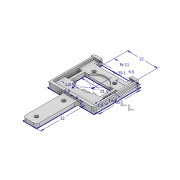
# Autodesk Inventor part: Intan_holder_test_main
Saved by Autodesk Inventor 2020 (Build 240168000, 168)
## iProperties
Created: 2020-07-20
Part Number: Intan_holder_test_main
Material: Generic
Document SubType Name: Modeling
Designer: Daniel
Density: 1 g/cm^3
Appearance: Default
Author: Daniel
Autodesk Inventor part; units mm, degrees
ref_plane "YZ Plane" through (0, 0, 0) normal (1, 0, 0) x (0, 1, 0)
ref_plane "XZ Plane" through (0, 0, 0) normal (0, 1, 0) x (-1, 0, 0)
ref_plane "XY Plane" through (0, 0, 0) normal (0, 0, 1) x (1, 0, 0)
sketch "Sketch1" plane through (0, 0, 0) normal (0, 1, 0) x (-1, 0, 0)
  line L0 (5, 16) -> (-5, 16)
  line L1 (-5, 16) -> (-5, -16)
  line L2 (-5, -16) -> (5, -16)
  line L3 (5, -16) -> (5, 16)
  line L4 (5, 16) -> (-5, -16) construction
  line L5 (-5, 16) -> (5, -16) construction
  line L6 (15.05, -16) -> (-15.05, -16)
  line L7 (-15.05, -16) -> (-15.05, -46.1)
  line L8 (-15.05, -46.1) -> (15.05, -46.1)
  line L9 (15.05, -46.1) -> (15.05, -16)
  line L10 (15.05, -16) -> (-15.05, -46.1) construction
  line L11 (-15.05, -16) -> (15.05, -46.1) construction
  line L12 (-17.05, -48.1) -> (-17.05, -14)
  line L13 (-17.05, -14) -> (17.05, -14)
  line L14 (17.05, -14) -> (17.05, -48.1)
  line L15 (17.05, -48.1) -> (-17.05, -48.1)
  line L16 (-11, -43.6) -> (11, -43.6)
  line L17 (10.55, -34.9) -> (-10.55, -34.9)
  line L18 (10.55, -24.8) -> (-10.55, -24.8)
  line L19 (10.55, -34.9) -> (-10.55, -34.9) construction
  line L20 (-10.55, -34.9) -> (-10.55, -24.8) construction
  line L21 (-10.55, -24.8) -> (10.55, -24.8)
  line L22 (10.55, -24.8) -> (10.55, -34.9) construction
  line L23 (10.55, -34.9) -> (-10.55, -24.8) construction
  line L24 (-10.55, -34.9) -> (10.55, -24.8) construction
  line L25 (10.55, -24.8) -> (10.55, -34.9)
  line L26 (-10.55, -24.8) -> (-10.55, -34.9)
  line L27 (-11, -43.6) -> (-11, -48.1)
  line L28 (11, -43.6) -> (11, -48.1)
  line L29 (15.05, -24.8) -> (12.35, -24.8)
  line L30 (12.35, -24.8) -> (12.35, -34.9)
  line L31 (12.35, -34.9) -> (15.05, -34.9)
  line L32 (15.05, -34.9) -> (15.05, -24.8)
  line L33 (-15.05, -24.8) -> (-12.35, -24.8)
  line L34 (-12.35, -24.8) -> (-12.35, -34.9)
  line L35 (-12.35, -34.9) -> (-15.05, -34.9)
  line L36 (-15.05, -34.9) -> (-15.05, -24.8)
  point P0 (0, 0)
  point P1 (0, -31.05)
  point P2 (0, 0)
  point P3 (0, -31.05)
  point P4 (0, -29.85)
  point P5 (0, -29.85)
  point P6 (0, -31.05)
  point P7 (5, -14)
  point P8 (-5, -14)
  point P9 (5, -16)
  point P10 (-5, -16)
  point P11 (-11, -46.1)
  point P12 (11, -46.1)
  point P13 (-15.05, -34.9)
  dimension "d19" = 10
  dimension "d20" = 32
  dimension "d23" = 30.1
  dimension "d24" = 30.1
  dimension "d26" = 2
  dimension "d29" = 4.5
  dimension "d31" = 8.8
  dimension "d32" = 21.1
  dimension "d33" = 10.1
  dimension "d37" = 22
  dimension "d38" = 11
  dimension "d132" = 1.8
  dimension "d133" = 1.8
  constraints: 74 end point, 12 parallel, 11 perpendicular, 10 midpoint, 7 point on line, 5 collinear, 5 horizontal, 2 vertical alignment, 3 other
  measures "d19" distance of L2.end L1.end
  measures "d20" distance of L1.end L0.end
  measures "d23" distance of L8.end L7.end
  measures "d24" distance of L7.end L6.end
  measures "d26" distance between parallel lines of L7 L12
  measures "d29" distance between parallel lines of L15 L16
  measures "d31" distance between parallel lines of L6 L18
  measures "d32" distance of L18.start L18.end
  measures "d33" distance of L18.end L19.end
  measures "d37" distance between parallel lines of L27 L28
  measures "d38" distance from line of point (0, -31.05) L28
  measures "d132" distance between parallel lines of L22 L30
  measures "d133" distance between parallel lines of L20 L34
extrude "Base" add sketch "Sketch1" along normal blind 2.6 contours L3 L13 L1 L0 | L3 L2 L1 L13 | L6 L9 L29 L30 L31 L8 L28 L16 L27 L7 L35 L34 L33 L2
extrude "Adaptor board recess" add sketch "Sketch1" along normal blind 4.2 contours L13 L14 L15 L28 L8 L9 L6 L3 | L3 L2 L1 L13 | L1 L6 L7 L8 L27 L15 L12 L13
sketch "Sketch3" plane through (0, 2.6, 0) normal (0, 1, 0) x (1, 0, 0)
  circle A0 centre (0, 31.05) radius 8.75
  line L0 (15.05, 16) -> (-15.05, 16) projected
  line L1 (-15.05, 16) -> (15.05, 16) projected
  line L2 (15.05, 34.9) -> (15.05, 46.1) projected
  line L3 (15.05, 46.1) -> (11, 46.1) projected
  line L4 (11, 46.1) -> (11, 43.6) projected
  line L5 (11, 43.6) -> (-11, 43.6) projected
  line L6 (-11, 43.6) -> (-11, 46.1) projected
  line L7 (-11, 46.1) -> (-15.05, 46.1) projected
  line L8 (-15.05, 46.1) -> (-15.05, 34.9) projected
  line L9 (10.55, 34.9) -> (10.55, 24.8) projected
  line L10 (10.55, 24.8) -> (-10.55, 24.8) projected
  line L11 (-10.55, 24.8) -> (-10.55, 34.9) projected
  line L12 (-10.55, 34.9) -> (10.55, 34.9) projected
  line L13 (15.05, 16) -> (15.05, 24.8) projected
  line L14 (15.05, 24.8) -> (12.35, 24.8) projected
  line L15 (12.35, 24.8) -> (12.35, 34.9) projected
  line L16 (12.35, 34.9) -> (15.05, 34.9) projected
  line L17 (-15.05, 34.9) -> (-12.35, 34.9) projected
  line L18 (-12.35, 34.9) -> (-12.35, 24.8) projected
  line L19 (-12.35, 24.8) -> (-15.05, 24.8) projected
  line L20 (-15.05, 24.8) -> (-15.05, 16) projected
  point P0 (0, 0)
  point P1 (0, 16)
  point P2 (-17.25, 14.5)
  point P3 (17.25, 14.5)
  point P4 (-9.5909, 26.1961)
  point P5 (9.5909, 26.1961)
  point P6 (6.1237, 24.8)
  point P7 (-6.1237, 24.8)
  point P8 (7.8575, 34.9)
  point P9 (9.5909, 31.858)
  point P10 (-9.5909, 31.858)
  point P11 (-7.8575, 34.9)
  dimension "d39" = 17.5
  constraints: 1 centre point, 1 coincident, 1 midpoint, 1 vertical alignment
  measures "d39" diameter of A0
extrude "EIB recess" cut sketch "Sketch3" against normal blind 1 contours L12 A0 | A0 L10
sketch "Sketch4" plane through (0, 2.6, 0) normal (0, 1, 0) x (1, 0, 0)
  circle A0 centre (7.5, 38.6) radius 1.3
  circle A1 centre (-7.5, 38.6) radius 1.3
  line L0 (5.9412, 41.3) -> (9.0588, 41.3)
  line L1 (9.0588, 41.3) -> (10.6177, 38.6)
  line L2 (10.6177, 38.6) -> (9.0588, 35.9)
  line L3 (9.0588, 35.9) -> (5.9412, 35.9)
  line L4 (5.9412, 35.9) -> (4.3823, 38.6)
  line L5 (4.3823, 38.6) -> (5.9412, 41.3)
  line L6 (-10.6177, 38.6) -> (-9.0588, 41.3)
  line L7 (-9.0588, 41.3) -> (-5.9412, 41.3)
  line L8 (-5.9412, 41.3) -> (-4.3823, 38.6)
  line L9 (-4.3823, 38.6) -> (-5.9412, 35.9)
  line L10 (-5.9412, 35.9) -> (-9.0588, 35.9)
  line L11 (-9.0588, 35.9) -> (-10.6177, 38.6)
  line L12 (11, 43.6) -> (-11, 43.6) construction
  point P0 (0, 0)
  dimension "d42" = 2.6
  dimension "d43" = 2.6
  dimension "d45" = 15
  dimension "d46" = 7.5
  dimension "d57" = 5.4
  dimension "d58" = 5.4
  dimension "d127" = 2.3
  constraints: 24 end point, 2 centre point, 2 coincident, 2 horizontal, 1 horizontal alignment, 26 other
  measures "d42" diameter of A0
  measures "d43" diameter of A1
  measures "d45" distance of A1.centre A0.centre
  measures "d46" horizontal distance of point (0, 0) A1.centre
  measures "d57" distance between parallel lines of L3 L0
  measures "d58" distance between parallel lines of L10 L7
  measures "d127" distance between parallel lines of L12 L7
extrude "Electrode mount holes" cut sketch "Sketch4" against normal through all contours A0 | A1
sketch "Sketch5" plane through (0, 2.6, 0) normal (0, 1, 0) x (1, 0, 0)
  circle A0 centre (0, 9) radius 1.3
  circle A1 centre (0, -11) radius 1.3
  line L0 (-17.05, 14) -> (17.05, 14) construction
  line L1 (-5, -16) -> (5, -16) construction
  line L2 (0, -16) -> (0, 14) construction
  point P0 (0, 0)
  dimension "d49" = 2.6
  dimension "d50" = 2.6
  dimension "d51" = 20
  dimension "d52" = 5
  constraints: 2 centre point, 2 end point, 2 midpoint, 1 point on line, 1 vertical alignment
  measures "d49" diameter of A0
  measures "d50" diameter of A1
  measures "d51" distance of A0.centre A1.centre
  measures "d52" distance from line of L0 A0.centre
extrude "Stick mount holes" cut sketch "Sketch5" against normal through all
sketch "Sketch6" plane through (17.05, 0, -14) normal (0, 0, -1) x (-1, 0, 0)
  line L0 (34.1, 4.2) -> (0, 4.2) construction
  line L1 (0, 0) -> (0, 4.2) construction
  line L2 (0, 4.2) -> (0, 2.2)
  line L3 (1, 2.2) -> (0, 2.2)
  line L4 (1, 2.2) -> (1.3, 2.5)
  line L5 (1, 2.2) -> (1.4243, 2.2) construction
  line L6 (1.3, 2.5) -> (0.7, 3.1)
  line L7 (1.3, 2.5) -> (2.1485, 2.5) construction
  line L8 (0.7, 3.1) -> (0.7, 4.2)
  line L9 (0, 4.2) -> (6.05, 4.2) construction
  line L10 (0, 4.2) -> (0.7, 4.2)
  line L11 (0.85, 4.35) -> (0.85, 3.1621)
  line L12 (0.85, 3.1621) -> (1.5121, 2.5)
  line L13 (1.5121, 2.5) -> (1.0621, 2.05)
  line L14 (1.0621, 2.05) -> (-0.15, 2.05)
  line L15 (-0.15, 2.05) -> (-0.15, 4.35)
  line L16 (-0.15, 4.35) -> (0.85, 4.35)
  point P0 (17.05, 0)
  dimension "d59" = 45
  dimension "d63" = 135
  dimension "d65" = 1
  dimension "d66" = 2
  dimension "d67" = 0.3
  dimension "d68" = 0.3
  dimension "d77" = 0.15
  constraints: 28 end point, 2 equal length, 2 horizontal, 2 perpendicular, 2 point on line, 1 collinear, 5 other
  measures "d59" angle of L5 L4
  measures "d63" angle of L7 L6
  measures "d65" distance from line of L1 L3.start
  measures "d66" distance from line of L0.end L3
  measures "d67" horizontal distance of L4.end L3.start
  measures "d68" distance from line of L3.start L8
  measures "d77" distance between parallel lines of L8 L11
extrude "Extrusion6" cut sketch "Sketch6" along normal blind 32 contours L10 L8 L6 L4 L3 L2 | L11 L12 L13 L14 L15 L16
mirror "Mirror1" about plane through (0, 0, 0) normal (1, 0, 0) of "Extrusion6"
fillet "Fillet3" radius 2 4 edges at (17.05, 2.1, -48.1) (17.05, 1.025, -14) (-17.05, 2.1, -48.1) (-17.05, 1.025, -14)
sketch "Sketch7" plane through (11, 0, -14) normal (0, 0, -1) x (-1, 0, 0)
  line L0 (-6.05, 2.2004) -> (-6.05, 10.15)
  line L1 (-6.05, 10.15) -> (11, 10.15)
  line L2 (-4.05, 4.2) -> (0, 4.2) construction
  line L3 (-4.05, 9.15) -> (11, 9.15)
  line L4 (11, 10.15) -> (11, 9.15)
  line L5 (11, -2.03) -> (11, 12.18) construction
  line L6 (-4.5379, 2.5) -> (-4.9879, 2.05)
  line L7 (-5.2, 3.1621) -> (-4.5379, 2.5)
  line L8 (-5.2, 4.2) -> (-5.2, 3.1621)
  line L9 (-4.7503, 2.5003) -> (-5.0502, 2.2004)
  line L10 (-5.0502, 2.2004) -> (-6.05, 2.2004)
  line L11 (-5.35, 4.05) -> (-5.35, 3.1)
  line L12 (-5.35, 3.1) -> (-4.7503, 2.5003)
  line L13 (-4.05, 9.15) -> (-4.05, 4.35)
  line L14 (-4.05, 2.6) -> (-4.05, 4.2) construction
  line L15 (-4.05, 4.35) -> (-5.35, 4.35)
  line L16 (-5.35, 4.35) -> (-5.35, 4.05)
  line L17 (-5.2, 3.1621) -> (-5.2, 4.2) construction
  line L18 (-4.5379, 2.5) -> (-5.2, 3.1621) construction
  line L19 (-4.9879, 2.05) -> (-4.5379, 2.5) construction
  line L20 (-6.05, 2.05) -> (-4.9879, 2.05) construction
  line L21 (-5.2, 4.2) -> (-4.05, 4.2) construction
  line L22 (-6.05, 0) -> (-6.05, 2.05) construction
  point P0 (11, 0)
  point P1 (-6.05, 4.2)
  dimension "d76" = 1
  dimension "d78" = 0.15
  dimension "d82" = 4.8
  dimension "d135" = 0.15
  dimension "d136" = 0.1504
  dimension "d137" = 0.1504
  constraints: 28 end point, 4 collinear, 3 point on line, 2 perpendicular, 2 vertical, 1 coincident, 1 horizontal, 3 other
  measures "d76" distance from line of L1 L3.start
  measures "d78" distance between parallel lines of L7 L12
  measures "d82" distance of L3.start L13.end
  measures "d135" distance between parallel lines of L21 L15
  measures "d136" distance between parallel lines of L6 L9
  measures "d137" distance between parallel lines of L20 L10
extrude "Extrusion7" add sketch "Sketch7" along normal blind 31.85 separate body
mirror "Mirror2" about plane through (0, 9.15, -14) normal (-1, 0, 0) of "Extrusion7" bodies 2
sketch "Sketch8" plane through (11, 0, -14) normal (0, 0, 1) x (-1, 0, 0)
  line L0 (27.35, -4.35) -> (26.05, -4.35) construction
  line L1 (22, 0) -> (22, -4.2) construction
  line L2 (0, 0) -> (0, -4.2) construction
  line L3 (-4.05, -9.15) -> (26.05, -9.15) construction
  line L4 (-4.05, -4.35) -> (-4.05, -9.15) construction
  line L5 (26.05, -4.35) -> (26.05, -9.15) construction
  line L6 (26.05, -9.15) -> (-4.05, -9.15)
  line L7 (-4.05, -9.15) -> (-4.05, -4.35)
  line L8 (-4.05, -4.35) -> (26.05, -4.35)
  line L9 (26.05, -4.35) -> (26.05, -9.15)
  line L10 (16.05, -9.15) -> (16.05, -4.35)
  line L11 (0, -4.2) -> (-4.05, -4.2) construction
  line L12 (5.95, -9.15) -> (5.95, -4.35)
  point P0 (11, 0)
  dimension "d149" = 10
  dimension "d150" = 10
  constraints: 13 end point, 4 point on line, 3 perpendicular, 2 parallel, 1 horizontal
  measures "d149" distance between parallel lines of L4 L12
  measures "d150" distance between parallel lines of L5 L10
extrude "Extrusion8" add sketch "Sketch8" against normal blind 2 contours L6 L10 L8 L9 | L6 L7 L8 L12 bodies 2
sketch "Sketch10" plane through (11, 0, -14) normal (0, 0, -1) x (-1, 0, 0)
  line L0 (-6.05, 5.9324) -> (-6.55, 5.0664)
  line L1 (-6.55, 5.0664) -> (-6.55, 3.0664)
  line L2 (-6.55, 3.0664) -> (-6.05, 2.2004)
  line L3 (-6.05, 2.2004) -> (-6.05, 5.9324)
  line L4 (-6.05, 10.15) -> (-6.05, 2.2004) construction
  point P0 (11, 0)
  dimension "d95" = 2
  dimension "d138" = 150
  dimension "d141" = 150
  dimension "d142" = 0.5
  constraints: 8 end point, 1 coincident, 1 point on line
  measures "d95" distance of L0.end L1.end
  measures "d138" angle of L1 L0
  measures "d141" angle of L1 L2
  measures "d142" distance between parallel lines of L3 L1
extrude "Extrusion10" add sketch "Sketch10" along normal up to surface (31.85 mm away) bodies 2
mirror "Mirror3" about plane through (0, 0, 0) normal (1, 0, 0) of "Extrusion10" bodies 2
sketch "Sketch13" plane through (11, 0, -45.85) normal (0, 0, -1) x (-1, 0, 0)
  line L0 (-4.7503, 2.5003) -> (-5.35, 3.1) construction
  line L1 (-5.35, 3.1) -> (-5.35, 4.35) construction
  line L2 (-5.35, 4.35) -> (-4.05, 4.35) construction
  line L3 (-4.05, 4.35) -> (-4.05, 9.15) construction
  line L4 (-4.05, 9.15) -> (26.05, 9.15) construction
  line L5 (26.05, 4.35) -> (26.05, 9.15) construction
  line L6 (27.35, 4.35) -> (26.05, 4.35) construction
  line L7 (27.35, 3.1) -> (27.35, 4.35) construction
  line L8 (26.7503, 2.5003) -> (27.35, 3.1) construction
  line L9 (27.0502, 2.2004) -> (26.7503, 2.5003) construction
  line L10 (28.05, 2.2004) -> (27.0502, 2.2004) construction
  line L11 (28.05, 2.2004) -> (28.55, 3.0664) construction
  line L12 (28.55, 3.0664) -> (28.55, 5.0664) construction
  line L13 (28.55, 5.0664) -> (28.05, 5.9324) construction
  line L14 (28.05, 10.15) -> (28.05, 5.9324) construction
  line L15 (-6.05, 10.15) -> (28.05, 10.15) construction
  line L16 (-6.05, 10.15) -> (-6.05, 5.9324) construction
  line L17 (-6.55, 5.0664) -> (-6.05, 5.9324) construction
  line L18 (-6.55, 3.0664) -> (-6.55, 5.0664) construction
  line L19 (-6.05, 2.2004) -> (-6.55, 3.0664) construction
  line L20 (-6.05, 2.2004) -> (-5.0502, 2.2004) construction
  line L21 (-5.0502, 2.2004) -> (-4.7503, 2.5003) construction
  line L22 (-6.05, 10.15) -> (-6.05, 5.9324) construction
  line L23 (-6.05, 10.15) -> (-4.05, 10.15)
  line L24 (-4.05, 10.15) -> (-4.05, 4.35)
  line L25 (-4.05, 4.35) -> (-6.05, 4.35)
  line L26 (-6.05, 4.35) -> (-6.05, 10.15)
  line L27 (26.05, 4.35) -> (26.05, 9.15) construction
  line L28 (28.05, 10.15) -> (26.05, 10.15)
  line L29 (26.05, 10.15) -> (26.05, 4.35)
  line L30 (26.05, 4.35) -> (28.05, 4.35)
  line L31 (28.05, 4.35) -> (28.05, 10.15)
  line L32 (-4.05, 10.15) -> (26.05, 10.15)
  line L33 (26.05, 10.15) -> (26.05, 7.85)
  line L34 (26.05, 7.85) -> (-4.05, 7.85)
  line L35 (-4.05, 7.85) -> (-4.05, 10.15)
  line L36 (0, 0) -> (0, 4.2) construction
  line L37 (22, 0) -> (22, 4.2) construction
  line L38 (-4.05, 4.35) -> (0, 4.35)
  line L39 (0, 4.35) -> (0, 7.85)
  line L40 (27.35, 4.35) -> (26.05, 4.35) construction
  line L41 (26.05, 4.35) -> (22, 4.35)
  line L42 (22, 4.35) -> (22, 7.85)
  point P0 (11, 0)
  point P1 (26.05, 10.15)
  dimension "d151" = 3.5
  constraints: 32 end point, 6 parallel, 5 perpendicular, 4 horizontal, 4 point on line, 2 collinear
  measures "d151" distance between parallel lines of L34 L38
extrude "Extrusion13" add sketch "Sketch13" along normal blind 2 bodies 2
fillet "Fillet8" radius 2 4 edges at (11, 7.85, -46.85) (-11, 7.85, -46.85) (-5.05, 9.15, -15) (5.05, 9.15, -15)
fillet "Fillet4" radius 2 8 edges at (-17.05, 8.0412, -14) (17.05, 8.0412, -14) (17.55, 4.0664, -14) (17.3, 5.4994, -14) (-17.3, 5.4994, -14) (-17.55, 4.0664, -14) (-17.05, 7.25, -47.85) (17.05, 7.25, -47.85)
fillet "Fillet9" radius 2 2 edges at (-17.05, 5.1412, -45.85) (17.05, 5.1412, -45.85)
chamfer "Chamfer1" distance 2 angle 45 8 edges at (-17.05, 10.15, -30.925) (-16.4642, 10.15, -47.2642) (0, 10.15, -47.85) (16.4642, 10.15, -47.2642) (17.05, 10.15, -30.925) (16.4642, 10.15, -14.5858) (0, 10.15, -14) (-16.4642, 10.15, -14.5858)
fillet "Fillet1" radius 2 4 edges at (5, 1.3, 16) (-5, 1.3, 16) (-5, 1.3, -14) (5, 1.3, -14)
sketch "Sketch11" plane through (0, 0, 0) normal (0, -1, 0) x (1, 0, 0)
  line L0 (-9.05, -24.8) -> (-9.05, -27.3)
  line L1 (-9.05, -27.3) -> (-10.55, -28.8)
  line L2 (-10.55, -24.8) -> (-10.55, -34.9) projected
  line L3 (10.55, -24.8) -> (-10.55, -24.8) projected
  line L4 (-10.55, -28.6586) -> (-9.15, -27.2586)
  line L5 (-9.15, -27.2586) -> (-9.15, -23.3)
  line L6 (-6.1237, -24.8) -> (6.1237, -24.8) construction
  line L7 (0, -24.8) -> (0, -33.4)
  line L8 (9.05, -24.8) -> (9.05, -27.3)
  line L9 (9.05, -27.3) -> (10.55, -28.8)
  line L10 (10.55, -24.8) -> (10.55, -34.9)
  line L11 (10.55, -28.6586) -> (9.15, -27.2586)
  line L12 (9.15, -27.2586) -> (9.15, -23.3)
  point P0 (0, 0)
  point P1 (9.15, -24.8)
  point P2 (-9.15, -24.8)
  dimension "d128" = 135
  dimension "d129" = 2.5
  dimension "d130" = 1.5
  dimension "d131" = 0.1
  constraints: 20 end point, 7 symmetric about line, 5 point on line, 2 vertical, 1 midpoint, 1 other
  measures "d128" angle of L0 L1
  measures "d129" distance of L0.start L0.end
  measures "d130" horizontal distance of L0.end L1.end
  measures "d131" distance between parallel lines of L1 L4
extrude "Extrusion11" add sketch "Sketch11" against normal blind 0.5 contours L5 L4 L2 L3 | L10 L11 L12 L3 bodies 1
fillet "Fillet6" radius 0.5 8 edges at (12.35, 1.3, -24.8) (12.35, 1.3, -34.9) (-12.35, 1.3, -34.9) (-12.35, 1.3, -24.8) (15.05, 1.3, -24.8) (15.05, 1.3, -34.9) (-15.05, 1.3, -24.8) (-15.05, 1.3, -34.9)
sketch "Sketch12" plane through (0, 2.6, 0) normal (0, 1, 0) x (1, 0, 0)
  line L0 (-6.1237, 24.8) -> (-10.55, 24.8) construction
  line L1 (-7.41, 24.8) -> (-1.41, 24.8)
  line L2 (-1.41, 24.8) -> (-1.41, 22.3)
  line L3 (-1.41, 22.3) -> (-7.41, 22.3)
  line L4 (-7.41, 22.3) -> (-7.41, 24.8)
  line L5 (-1.41, 22.3) -> (-7.41, 24.8) construction
  line L6 (-7.41, 22.3) -> (-1.41, 24.8) construction
  line L7 (-9.15, 24.8) -> (-9.15, 27.2586) construction
  point P0 (0, 0)
  point P1 (-4.41, 23.55)
  dimension "d143" = 4.74
  dimension "d144" = 2.5
  dimension "d145" = 6
  constraints: 12 end point, 2 parallel, 1 horizontal, 1 midpoint, 1 perpendicular, 1 point on line
  measures "d143" distance from line of L7 point (-4.41, 23.55)
  measures "d144" distance of L3.end L1.start
  measures "d145" distance between parallel lines of L2 L4
extrude "Extrusion12" cut sketch "Sketch12" against normal through all bodies 1
fillet "Fillet7" radius 0.5 2 edges at (-1.41, 1.3, -22.3) (-7.41, 1.3, -22.3)
equation "\"d38\" = 0.5 * d37"
equation "\"d43\" = d42"
equation "\"d46\" = 0.5 * d45"
equation "\"d58\" = d57"
equation "\"d50\" = d49"
body "Solid1"
body "Solid2"
